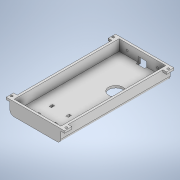
# Autodesk Inventor part: TOP_HOLDER_ENGER-2200
Saved by Autodesk Inventor 2022 (Build 260153000, 153)
## iProperties
Created: 2022-11-10
Part Number: TOP_HOLDER_ENGER-2200
Material: Generic
Document SubType Name: Modeling
Designer: udhay
Density: 1 g/cm^3
Appearance: Default
Author: udhay
## iProperties of the stored document TOP_HOLDER_ENGER-2200_3DPrint.ipt
Created: 2022-11-17
Part Number: TOP_HOLDER_ENGER-2200_3DPrint
Material: Generic
Document SubType Name: Modeling
Designer: udhay
Density: 1 g/cm^3
Appearance: Default
Author: udhay
Autodesk Inventor part; units mm, degrees
ref_plane "YZ Plane" through (0, 0, 0) normal (1, 0, 0) x (0, 1, 0)
ref_plane "XZ Plane" through (0, 0, 0) normal (0, 1, 0) x (-1, 0, 0)
ref_plane "XY Plane" through (0, 0, 0) normal (0, 0, 1) x (1, 0, 0)
sketch "Sketch1" plane through (0, 0, 0) normal (0, 1, 0) x (-1, 0, 0)
  line L0 (0, 0) -> (70, 0)
  line L1 (70, 0) -> (70, -150)
  line L2 (70, -150) -> (0, -150)
  line L3 (0, -150) -> (0, 0)
  dimension "d0" = 70
  dimension "d1" = 150
  constraints: 8 end point, 2 parallel, 1 horizontal, 1 perpendicular
  measures "d0" distance of L1.end L2.end
  measures "d1" distance of L0.end L1.end
extrude "Extrusion1" add sketch "Sketch1" along normal blind 18
sketch "Sketch2" plane through (0, 18, 0) normal (0, 1, 0) x (1, 0, 0)
  line L0 (0, 0) -> (-3, 0)
  line L1 (-3, 0) -> (-3, 3)
  line L2 (-3, 3) -> (0, 3)
  line L3 (0, 3) -> (0, 0)
  line L4 (0, 150) -> (-70, 150) projected
  line L5 (-70, 150) -> (-67, 150)
  line L6 (-67, 150) -> (-67, 147)
  line L7 (-67, 147) -> (-70, 147)
  line L8 (-70, 147) -> (-70, 150)
  line L9 (-67, 147) -> (-3, 147)
  line L10 (-3, 147) -> (-3, 3)
  line L11 (-3, 3) -> (-67, 3)
  line L12 (-67, 3) -> (-67, 147)
  dimension "d4" = 3
  dimension "d5" = 3
  dimension "d6" = 3
  dimension "d7" = 3
  constraints: 24 end point, 6 parallel, 3 horizontal, 3 perpendicular
  measures "d4" distance of L1.end L2.end
  measures "d5" distance of L0.end L1.end
  measures "d6" distance of L6.end L7.end
  measures "d7" distance of L5.end L6.end
extrude "Extrusion2" cut sketch "Sketch2" against normal blind 15 contours L11 L12 L9 L10
sketch "Sketch3" plane through (0, 0, 0) normal (0, -1, 0) x (1, 0, 0)
  circle A0 centre (-21.826, -97.2538) radius 9.7861
  point P0 (0, 0)
  constraints: 1 centre point
sketch "Sketch12" plane through (0, 18, 0) normal (0, 1, 0) x (1, 0, 0)
  line L0 (-70, 150) -> (-70, 0) projected
  line L1 (-70, 0) -> (-75, 0)
  line L2 (-75, 0) -> (-75, 10)
  line L3 (-75, 10) -> (-70, 10)
  line L4 (-70, 10) -> (-70, 0)
  line L5 (-70, 0) -> (0, 0) projected
  line L6 (0, 0) -> (5, 0)
  line L7 (5, 0) -> (5, 10)
  line L8 (5, 10) -> (0, 10)
  line L9 (0, 10) -> (0, 0)
  line L10 (-70, 150) -> (-75, 150)
  line L11 (-75, 150) -> (-75, 140)
  line L12 (-75, 140) -> (-70, 140)
  line L13 (-70, 140) -> (-70, 150)
  line L14 (0, 150) -> (-70, 150) projected
  line L15 (0, 150) -> (5, 150)
  line L16 (5, 150) -> (5, 140)
  line L17 (5, 140) -> (0, 140)
  line L18 (0, 140) -> (0, 150)
  dimension "d47" = 5
  dimension "d48" = 10
  dimension "d49" = 5
  dimension "d50" = 10
  dimension "d51" = 5
  dimension "d52" = 10
  dimension "d53" = 10
  constraints: 32 end point, 8 parallel, 4 horizontal, 4 perpendicular, 1 point on line
  measures "d47" distance of L2.end L3.end
  measures "d48" distance of L1.end L2.end
  measures "d49" distance of L8.end L7.end
  measures "d50" distance of L7.end L6.end
  measures "d51" distance of L12.end L11.end
  measures "d52" distance of L11.end L10.end
  measures "d53" distance of L15.end L16.end
extrude "Extrusion10" add sketch "Sketch12" against normal blind 3
sketch "Sketch13" plane through (0, 18, 0) normal (0, 1, 0) x (1, 0, 0)
  line L0 (5, 10) -> (5, 0) projected
  line L1 (5, 10) -> (2.5, 10)
  line L2 (5, 5) -> (5, 10)
  circle A0 centre (2.5, 5) radius 1.5
  line L3 (0, 150) -> (5, 150) projected
  line L4 (5, 150) -> (2.5, 150)
  line L5 (5, 145) -> (5, 150)
  line L6 (-75, 150) -> (-70, 150) projected
  line L7 (-75, 150) -> (-72.8563, 150)
  line L8 (-75, 145) -> (-75, 150)
  line L9 (-75, 10) -> (-70, 10) projected
  line L10 (-75, 10) -> (-72.5, 10)
  line L11 (-75, 5) -> (-75, 10)
  circle A1 centre (-72.5, 5) radius 1.5
  circle A2 centre (2.5, 145) radius 1.5
  circle A3 centre (-72.8563, 144.7862) radius 1.5
  point P0 (0, 0)
  constraints: 16 end point, 4 centre point, 4 horizontal
extrude "Extrusion11" cut sketch "Sketch13" against normal blind 10
extrude "Extrusion12" cut sketch "Sketch3" against normal blind 10
sketch "Sketch14" plane through (0, 0, -150) normal (0, 0, -1) x (-1, 0, 0)
  line L0 (75, 18) -> (-5, 18) projected
  line L1 (75, 18) -> (35, 18)
  line L2 (75, 12.0072) -> (75, 18)
  line L3 (57.75, 7.8) -> (12.25, 7.8)
  line L4 (12.25, 7.8) -> (12.25, 28.2)
  line L5 (12.25, 28.2) -> (57.75, 28.2)
  line L6 (57.75, 28.2) -> (57.75, 7.8)
  line L7 (57.75, 7.8) -> (57.25, 7.8)
  line L8 (57.75, 8.3) -> (57.75, 7.8)
  circle A0 centre (55.9, 9.65) radius 1.35
  line L9 (54.05, 7.8) -> (54.55, 7.8)
  circle A1 centre (14.1, 9.65) radius 1.35
  line L10 (12.25, 8.3) -> (12.25, 7.8)
  point P0 (0, 0)
  dimension "d74" = 45.5
  dimension "d75" = 20.4
  constraints: 20 end point, 3 horizontal, 2 centre point, 2 parallel, 1 perpendicular
  measures "d74" distance of L4.end L5.end
  measures "d75" distance of L3.end L4.end
extrude "Extrusion13" cut sketch "Sketch14" against normal blind 10 contours A0 | A1
sketch "Sketch15" plane through (0, 0, 0) normal (0, -1, 0) x (1, 0, 0)
  line L0 (-3, -3) -> (-67, -3) projected
  line L1 (-67, -3) -> (-3, -3)
  line L2 (-3, -3) -> (-67, -3) projected
  line L3 (-67, -3) -> (-3, -3)
  line L4 (-3, -3) -> (-3, -13)
  line L5 (-67, -13) -> (-67, -3)
  line L6 (-67, -13) -> (-3, -13)
  point P0 (0, 0)
  constraints: 10 end point, 3 horizontal, 1 parallel, 1 perpendicular
sketch "Sketch16" plane through (0, 0, 0) normal (0, -1, 0) x (1, 0, 0)
  line L0 (-70, 0) -> (0, 0) projected
  line L1 (-70, 0) -> (-47, 0)
  line L2 (-70, -9.9091) -> (-70, 0)
  line L3 (0, 0) -> (-26, 0)
  line L4 (0, -9.0382) -> (0, 0)
  line L5 (-26, 0) -> (-36.5, 0)
  line L6 (-46.5, -38) -> (-26.5, -38)
  line L7 (-26.5, 38) -> (-46.5, 38)
  line L8 (-46.5, 0) -> (-26.5, 0)
  line L9 (-26.5, -10) -> (-46.5, -10)
  line L10 (-46.5, -10) -> (-46.5, 0)
  line L11 (-26.5, -38) -> (-26.5, -10)
  line L12 (-26.5, 0) -> (-26.5, 38)
  line L13 (-46.5, 38) -> (-46.5, 0)
  line L14 (-46.5, -10) -> (-46.5, -38)
  line L15 (-26.5, -29) -> (-26.5, -38)
  line L16 (-26.5, -10) -> (-23.5, -10)
  line L17 (-23.5, -10) -> (-23.5, -19)
  line L18 (-23.5, -19) -> (-26.5, -19)
  line L19 (-26.5, -19) -> (-26.5, -10)
  line L20 (-26.5, -38) -> (-23.5, -38)
  line L21 (-23.5, -38) -> (-23.5, -29)
  line L22 (-23.5, -29) -> (-26.5, -29)
  line L23 (-26.5, -29) -> (-26.5, -38)
  line L24 (-46.5, -38) -> (-49.5, -38)
  line L25 (-49.5, -38) -> (-49.5, -29)
  line L26 (-49.5, -29) -> (-46.5, -29)
  line L27 (-46.5, -29) -> (-46.5, -38)
  line L28 (-46.5, -10) -> (-49.5, -10)
  line L29 (-49.5, -10) -> (-49.5, -19)
  line L30 (-49.5, -19) -> (-46.5, -19)
  line L31 (-46.5, -19) -> (-46.5, -10)
  line L32 (-46.5, -38) -> (-49.5, -38)
  line L33 (-49.5, -38) -> (-49.5, -33.5)
  line L34 (-49.5, -33.5) -> (-46.5, -33.5)
  line L35 (-46.5, -33.5) -> (-46.5, -38)
  line L36 (-46.5, -19) -> (-49.5, -19)
  line L37 (-49.5, -19) -> (-49.5, -14.5)
  line L38 (-49.5, -14.5) -> (-46.5, -14.5)
  line L39 (-46.5, -14.5) -> (-46.5, -19)
  line L40 (-26.5, -38) -> (-23.5, -38)
  line L41 (-23.5, -38) -> (-23.5, -33.5)
  line L42 (-23.5, -33.5) -> (-26.5, -33.5)
  line L43 (-26.5, -33.5) -> (-26.5, -38)
  line L44 (-26.5, -19) -> (-23.5, -19)
  line L45 (-23.5, -19) -> (-23.5, -14.5)
  line L46 (-23.5, -14.5) -> (-26.5, -14.5)
  line L47 (-26.5, -14.5) -> (-26.5, -19)
  dimension "d91" = 20
  dimension "d97" = 3
  dimension "d98" = 9
  dimension "d99" = 3
  dimension "d100" = 9
  dimension "d101" = 3
  dimension "d102" = 9
  dimension "d103" = 9
  constraints: 94 end point, 22 parallel, 13 horizontal, 10 perpendicular, 4 midpoint, 1 point on line
  measures "d91" distance of L7.end L7.start
  measures "d97" distance of L17.end L18.end
  measures "d98" distance of L16.end L17.end
  measures "d99" distance of L22.end L21.end
  measures "d100" distance of L21.end L20.end
  measures "d101" distance of L25.end L26.end
  measures "d102" distance of L24.end L25.end
  measures "d103" distance of L29.end L28.end
extrude "Extrusion15" cut sketch "Sketch15" against normal blind 10
extrude "Extrusion16" cut sketch "Sketch16" against normal blind 10 contours L24 L25 L34 L14 | L11 L42 L21 L20 | L30 L29 L38 L14 | L11 L46 L17 L18
sketch "Sketch18" plane through (0, 0, 0) normal (0, -1, 0) x (1, 0, 0)
  line L0 (-70, -140) -> (-70, -150) projected
  line L1 (-70, -150) -> (-35, -150)
  line L2 (-70, -148.5164) -> (-70, -150)
  line L3 (-29.25, -156) -> (-29.25, -144)
  line L4 (-29.25, -144) -> (-40.75, -144)
  line L5 (-40.75, -144) -> (-40.75, -156)
  line L6 (5, -150) -> (-75, -150) projected
  line L7 (-40.75, -150) -> (-29.25, -150)
  point P0 (0, 0)
  dimension "d107" = 11.5
  dimension "d108" = 12
  constraints: 12 end point, 2 midpoint, 2 point on line, 1 horizontal, 1 parallel
  measures "d107" distance of L4.end L3.end
  measures "d108" distance of L3.end L3.start
extrude "Extrusion17" cut sketch "Sketch18" against normal blind 10
fillet "Face Fillet1" radius 5.5 1 edges at (0, 0, -75)
fillet "Face Fillet2" radius 5.5 1 edges at (-70, 0, -75)
body "Solid1"
